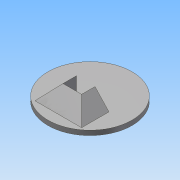
# Autodesk Inventor part: Membran_Platte
Saved by Autodesk Inventor 2015 (Build 190159000, 159)
## iProperties
Created: 2015-09-01
Part Number: Membran_Platte
Material: Stahl
Document SubType Name: Modeling
Designer: Johann
Density: 7.85 g/cm^3
Appearance: Stahl
Author: Johann
Autodesk Inventor part; units mm, degrees
ref_plane "YZ Plane" through (0, 0, 0) normal (1, 0, 0) x (0, 1, 0)
ref_plane "XZ Plane" through (0, 0, 0) normal (0, 1, 0) x (-1, 0, 0)
sketch "Skizze1" plane through (0, 0, 0) normal (0, 0, 1) x (1, 0, 0)
  circle A0 centre (0, 0) radius 9
  dimension "d0" = 18
  constraints: 1 centre point, 1 coincident
  measures "d0" diameter of A0
extrude "Extrusion1" add sketch "Skizze1" along normal mid plane 1
sketch "Skizze2" plane through (0, 0, 0.5) normal (0, 0, 1) x (1, 0, 0)
  line L0 (-5.3, -0.925) -> (-2, -0.925)
  line L1 (-2, -0.925) -> (-2, -3.8)
  line L2 (-2, -3.8) -> (2, -3.8)
  line L3 (2, -3.8) -> (2, -0.925)
  line L4 (2, -0.925) -> (5.3, -0.925)
  line L5 (5.3, -0.925) -> (5.3, -7.1)
  line L6 (5.3, -7.1) -> (-5.3, -7.1)
  line L7 (-5.3, -7.1) -> (-5.3, -0.925)
  point P0 (0, 0)
  point P1 (0, -3.8)
  dimension "d3" = 4
  dimension "d4" = 2.875
  dimension "d5" = 3.3
  dimension "d6" = 3.3
  dimension "d17" = 3.8
  constraints: 16 end point, 5 perpendicular, 2 point on line, 1 collinear, 1 horizontal, 1 midpoint, 1 vertical, 1 vertical alignment
  measures "d3" distance of L1.end L2.end
  measures "d4" distance of L0.end L1.end
  measures "d5" distance of L0.start L0.end
  measures "d6" distance between parallel lines of L6 L2
  measures "d17" distance from line of point (0, 0) L2
extrude "Extrusion3" add sketch "Skizze2" along normal blind 3.3
ref_plane "Arbeitsebene3" through (0, 0, 0.5) normal (0, 0, 1) x (1, 0, 0)
sketch "Skizze5" plane through (0, 0, 0.5) normal (0, 0, 1) x (1, 0, 0)
  line L0 (-2, -0.925) -> (-2, -3.8) construction
  line L1 (-2, -3.8) -> (2, -3.8) construction
  line L2 (2, -3.8) -> (2, -0.925) construction
  line L3 (2, -0.925) -> (5.3, -0.925) construction
  line L4 (5.3, -0.925) -> (5.3, -7.1) construction
  line L5 (5.3, -7.1) -> (-5.3, -7.1) construction
  line L6 (-5.3, -7.1) -> (-5.3, -0.925) construction
  line L7 (-5.3, -0.925) -> (-2, -0.925) construction
  circle A0 centre (0, 0) radius 9 construction
  line L8 (-5.3, -0.925) -> (-5.3, 7.2739)
  line L9 (-5.3, 7.2739) -> (5.3, 7.2739)
  circle A1 centre (0, 0) radius 9 projected
  line L10 (5.3, 7.2739) -> (5.3, -0.925)
  line L11 (-5.3, -0.925) -> (5.3, -0.925)
  dimension "d26" = 8.1989
  constraints: 8 end point, 2 horizontal, 2 point on circle, 1 vertical, 2 other
  measures "d26" distance between parallel lines of L9 L11
extrude "Extrusion4" add sketch "Skizze5" along normal up to surface (3.3 mm away) contours L8 L9 L10 L11
chamfer "Fase1" distance 3.3 angle 45 3 edges at (0, -7.1, 3.8) (5.3, 0.087, 3.8) (-5.3, 0.087, 3.8)
chamfer "Fase2" distance 3.3 distance2 8.1989 1 edges at (0, 7.2739, 3.8) measured on face at (0.6667, 7.2739, 1.6)
equation "\"d6\" = d5"
equation "\"d28\" = d26"
